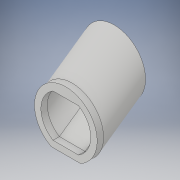
# Autodesk Inventor part: ramp bottom connect
Saved by Autodesk Inventor 2017 (Build 210142000, 142)
## iProperties
Created: 2018-03-06
Part Number: ramp bottom connect
Material: Generic
Document SubType Name: Modeling
Designer: braxtonwright
Density: 1 g/cm^3
Appearance: Default
Author: braxtonwright
Autodesk Inventor part; units mm, degrees
ref_plane "YZ Plane" through (0, 0, 0) normal (1, 0, 0) x (0, 1, 0)
ref_plane "XZ Plane" through (0, 0, 0) normal (0, 1, 0) x (-1, 0, 0)
ref_plane "XY Plane" through (0, 0, 0) normal (0, 0, 1) x (1, 0, 0)
sketch "Sketch1" plane through (0, 0, 0) normal (0, 0, 1) x (1, 0, 0)
  line L0 (-50.8, 84.6667) -> (50.8, 84.6667)
  line L1 (-50.8, -84.6667) -> (50.8, -84.6667)
  arc A0 (57.793, -110.0667) -> (-57.793, -110.0667) centre (0, 0) ccw
  arc A1 (-50.8, 84.6667) -> (-50.8, -84.6667) centre (0, 0) ccw
  arc A2 (50.8, -84.6667) -> (50.8, 84.6667) centre (0, 0) ccw
  line L2 (-57.793, -110.0667) -> (57.793, -110.0667)
  dimension "d0" = 169.3333
  dimension "d1" = 101.6
  dimension "d2" = 25.4
  constraints: 6 end point, 6 point on circle, 3 centre point, 3 horizontal, 2 coincident, 1 parallel
  measures "d0" distance between parallel lines of L1 L0
  measures "d1" distance of L0.start L0.end
  measures "d2" distance between parallel lines of L1 L2
ref_plane "Work Plane2" through (0, 0, 203.2) normal (0, 0, 1) x (1, 0, 0)
sketch "Sketch6" plane through (0, 0, 0) normal (1, 0, 0) x (0, 1, 0)
  line L0 (-110.0667, 0) -> (124.3169, 0) projected
  line L1 (-83.4784, 0) -> (-200.0291, 166.4517)
  point P0 (0, 0)
  dimension "d28" = 203.2
  dimension "d29" = 55
  constraints: 2 end point, 1 point on line
  measures "d28" distance of L1.start L1.end
  measures "d29" angle of L0 L1
sweep "ramp" add profiles "Sketch1" path "Sketch6" path curves L1
sketch "Sketch7" plane through (0, -116.5507, 166.4517) normal (0, 0, 1) x (1, 0, 0)
  arc A0 (-50.8, 84.6667) -> (-50.8, -84.6667) centre (0, 0) ccw projected
  arc A1 (57.793, -110.0667) -> (-57.793, -110.0667) centre (0, 0) ccw
  line L0 (50.8, -84.6667) -> (-50.8, -84.6667) projected
  line L1 (-50.8, -84.6667) -> (50.8, -84.6667)
  arc A2 (57.793, -110.0667) -> (-57.793, -110.0667) centre (0, 0) ccw projected
  line L2 (57.793, -110.0667) -> (-57.793, -110.0667)
  line L3 (50.8, 201.2174) -> (50.8, 84.6667) projected
  line L4 (-50.8, 84.6667) -> (50.8, 84.6667)
  arc A3 (-50.8, 84.6667) -> (-50.8, -84.6667) centre (0, 0) ccw
  arc A4 (50.8, -84.6667) -> (50.8, 84.6667) centre (0, 0) ccw
  point P0 (0, 116.5507)
  constraints: 6 end point, 6 point on circle, 3 centre point, 2 coincident, 1 collinear, 1 horizontal, 1 parallel
extrude "connection bottom" add sketch "Sketch7" along normal blind 25.4
body "Solid1"
